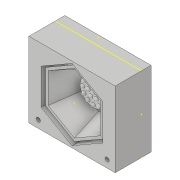
# Autodesk Inventor part: exploration1
Saved by Autodesk Inventor 2019 (Build 230136000, 136)
## iProperties
Created: 2020-02-16
Part Number: exploration1
Material: Generic
Document SubType Name: Modeling
Designer: Sandeep Shankar P
Density: 1 g/cm^3
Appearance: Default
Author: Sandeep Shankar P
Autodesk Inventor part; units mm, degrees
ref_plane "YZ Plane" through (0, 0, 0) normal (1, 0, 0) x (0, 1, 0)
sketch "Sketch1" plane through (0, 0, 0) normal (0, 0, 1) x (1, 0, 0)
  line L0 (0, 46.188) -> (40, 23.094)
  line L1 (40, 23.094) -> (40, -23.094)
  line L2 (40, -23.094) -> (0, -46.188)
  line L3 (0, -46.188) -> (-40, -23.094)
  line L4 (-40, -23.094) -> (-40, 23.094)
  line L5 (-40, 23.094) -> (0, 46.188)
  point P0 (0, 0)
  point P1 (0, 0)
  dimension "d0" = 80
  dimension "d1" = 80
  constraints: 12 end point, 1 coincident, 13 other
  measures "d0" distance between parallel lines of L3 L0
  measures "d1" distance between parallel lines of L1 L4
ref_plane "Work Plane1" through (0, 0, 50) normal (0, 0, 1) x (1, 0, 0)
sketch "Sketch2" plane through (0, 0, 50) normal (0, 0, 1) x (1, 0, 0)
  line L0 (0, -69.282) -> (-60, -34.641)
  line L1 (-60, -34.641) -> (-60, 34.641)
  line L2 (-60, 34.641) -> (0, 69.282)
  line L3 (0, 69.282) -> (60, 34.641)
  line L4 (60, 34.641) -> (60, -34.641)
  line L5 (60, -34.641) -> (0, -69.282)
  point P0 (0, 0)
  point P1 (0, 0)
  dimension "d3" = 120
  constraints: 12 end point, 1 coincident, 13 other
  measures "d3" distance between parallel lines of L2 L5
loft "Loft1" add profiles "Sketch1", "Sketch2"
sketch "Sketch3" plane through (0, 0, 50) normal (0, 0, 1) x (1, 0, 0)
  point P0 (0, 0)
shell "Shell2" thickness 5 removed faces 2 at (20, 11.547, 50) at (13.3333, 7.698, 0)
sketch "Sketch4" plane through (0, 0, 0) normal (0, 0, 1) x (1, 0, 0)
  circle A0 centre (0, 0) radius 28.0716
  constraints: 1 centre point, 1 coincident
extrude "Extrusion1" add sketch "Sketch4" along normal blind 10
sketch "Sketch5" plane through (0, 0, 0) normal (0, 0, -1) x (-1, 0, 0)
  circle A0 centre (0, 0) radius 2.5
  dimension "d34" = 5
  constraints: 1 centre point, 1 coincident
  measures "d34" diameter of A0
extrude "Extrusion2" cut sketch "Sketch5" against normal blind 5
sketch "Sketch6" plane through (0, 0, 10) normal (0, 0, 1) x (1, 0, 0)
  circle A0 centre (22.5, 0) radius 4
  circle A1 centre (0, 0) radius 28.0716 projected
  circle A2 centre (0, 0) radius 2.5 projected
  circle A3 centre (0, 0) radius 22.5
  circle A4 centre (19.4856, 11.25) radius 4
  circle A5 centre (11.25, 19.4856) radius 4
  circle A6 centre (0, 22.5) radius 4
  circle A7 centre (-11.25, 19.4856) radius 4
  circle A8 centre (-19.4856, 11.25) radius 4
  circle A9 centre (-22.5, 0) radius 4
  circle A10 centre (-19.4856, -11.25) radius 4
  circle A11 centre (-11.25, -19.4856) radius 4
  circle A12 centre (0, -22.5) radius 4
  circle A13 centre (11.25, -19.4856) radius 4
  circle A14 centre (19.4856, -11.25) radius 4
  circle A15 centre (0, 0) radius 11.25
  circle A16 centre (11.25, 0) radius 4.2356
  circle A17 centre (5.625, 9.7428) radius 4.2356
  circle A18 centre (-5.625, 9.7428) radius 4.2356
  circle A19 centre (-11.25, 0) radius 4.2356
  circle A20 centre (-5.625, -9.7428) radius 4.2356
  circle A21 centre (5.625, -9.7428) radius 4.2356
  circle A22 centre (0, 0) radius 4
  dimension "d15" = 8
  dimension "d16" = 22.5
  dimension "d19" = 360
  dimension "d23" = 360
  constraints: 19 centre point, 3 coincident, 2 horizontal alignment, 42 other
  measures "d15" diameter of A0
  measures "d16" distance of A1.centre A0.centre
extrude "Extrusion3" add sketch "Sketch6" along normal blind 4 contours A0 A3 | A3 A0 | A4 A3 | A3 A4 | A14 A3 | A3 A14 | A5 A3 | A3 A5 | A13 A3 | A3 A13 | A6 A3 | A3 A6 | A12 A3 | A3 A12 | A7 A3 | A3 A7 | A11 A3 | A3 A11 | A8 A3 | A3 A8 | A10 A3 | A3 A10 | A9 A3 | A3 A9 | A2 | A15 A16 | A15 A16 | A17 A15 | A15 A17 | A21 A15 | A15 A21 | A18 A15 | A15 A18 | A20 A15 | A15 A20 | A19 A15 | A15 A19 | A22
fillet "Fillet1" radius 4 19 edges at (7.25, 19.4856, 14) (15.4856, 11.25, 14) (18.5, 0, 14) (15.4856, -11.25, 14) (7.25, -19.4856, 14) (-4, -22.5, 14) (-15.25, -19.4856, 14) (-23.4856, -11.25, 14) (-26.5, 0, 14) (-23.4856, 11.25, 14) (-15.25, 19.4856, 14) (-4, 22.5, 14) (1.3894, 9.7428, 14) (7.0144, 0, 14) (1.3894, -9.7428, 14) (-9.8606, -9.7428, 14) (-15.4856, 0, 14) (-9.8606, 9.7428, 14) (-4, 0, 14)
sketch "Sketch7" plane through (0, 0, 0) normal (0, 0, -1) x (-1, 0, 0)
  line L0 (-90, -78.4325) -> (90, -78.4325)
  line L1 (90, -78.4325) -> (90, 78.4325)
  line L2 (90, 78.4325) -> (-90, 78.4325)
  line L3 (-90, 78.4325) -> (-90, -78.4325)
  line L4 (-90, -78.4325) -> (90, 78.4325) construction
  line L5 (90, -78.4325) -> (-90, 78.4325) construction
  circle A0 centre (0, 0) radius 2.5 projected
  circle A1 centre (0, 0) radius 2.49
  dimension "d30" = 180
  constraints: 12 end point, 2 midpoint, 2 parallel, 1 centre point, 1 coincident, 1 horizontal, 1 perpendicular
  measures "d30" distance between parallel lines of L1 L3
extrude "Extrusion4" add sketch "Sketch7" along normal blind 20 contours L3 L2 L1 L0
sketch "Sketch8" plane through (-60, -34.641, 50) normal (0, 0, 1) x (1, 0, 0)
  point P0 (60, 34.641)
sketch "Sketch9" plane through (0, 0, 0) normal (0, 0, 1) x (1, 0, 0)
  line L0 (-90, 78.4325) -> (90, 78.4325) projected
  point P0 (0, 0)
  point P1 (90, -78.4325)
sketch "Sketch10" plane through (0, 0, 0) normal (0, 0, 1) x (1, 0, 0)
  line L0 (90, -78.4325) -> (-90, -78.4325) projected
  line L1 (90, 78.4325) -> (90, -78.4325)
  line L2 (90, -78.4325) -> (-90, -78.4325)
  line L3 (-90, -78.4325) -> (-90, 78.4325)
  line L4 (-90, 78.4325) -> (90, 78.4325) projected
  line L5 (-90, 78.4325) -> (90, 78.4325)
  circle A0 centre (0, 0) radius 2.5 projected
  line L6 (64.4365, 37.2024) -> (64.4365, -37.2024)
  line L7 (64.4365, -37.2024) -> (0, -74.4049)
  line L8 (0, -74.4049) -> (-64.4365, -37.2024)
  line L9 (-64.4365, -37.2024) -> (-64.4365, 37.2024)
  line L10 (-64.4365, 37.2024) -> (0, 74.4049)
  line L11 (0, 74.4049) -> (64.4365, 37.2024)
  dimension "d33" = 156.865
  constraints: 20 end point, 2 collinear, 2 perpendicular, 1 coincident, 13 other
  measures "d33" distance between parallel lines of L0 L4
extrude "Extrusion5" add sketch "Sketch10" along normal blind 54.925 contours L0 L3 L4 L1
sketch "Sketch11" plane through (90, -78.4325, -20) normal (1, 0, 0) x (0, 0, -1)
  point P0 (-20, 78.4325)
sketch "Sketch12" plane through (-90, 78.4325, -20) normal (0, 1, 0) x (1, 0, 0)
  point P0 (90, -20)
ref_plane "Work Plane2" through (-90, 93.4325, -20) normal (0, 1, 0) x (1, 0, 0)
sketch "Sketch13" plane through (-90, 93.4325, -20) normal (0, 1, 0) x (1, 0, 0)
  point P0 (90, -20)
sketch "Sketch14" plane through (0, 0, 54.925) normal (0, 0, 1) x (1, 0, 0)
  circle A0 centre (73.3456, -62.6528) radius 4.253
  circle A1 centre (-70.3382, -62.6528) radius 4.3696
  point P0 (0, 0)
  constraints: 2 centre point
extrude "Extrusion6" cut sketch "Sketch14" against normal blind 75.0875
body "Solid1"
